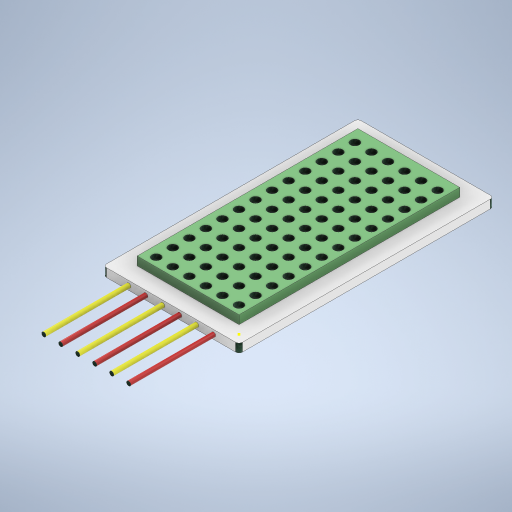
# Autodesk Inventor part: circuit
Saved by Autodesk Inventor 2024 (Build 280153000, 153)
## iProperties
Created: 2024-02-01
Part Number: circuit
Material: Generic
Document SubType Name: Modeling
Designer: RAHUL
Density: 1 g/cm^3
Appearance: Green Polished
Author: RAHUL
Autodesk Inventor part; units mm, degrees
ref_plane "YZ Plane" through (0, 0, 0) normal (1, 0, 0) x (0, 1, 0)
ref_plane "XZ Plane" through (0, 0, 0) normal (0, 1, 0) x (-1, 0, 0)
ref_plane "XY Plane" through (0, 0, 0) normal (0, 0, 1) x (1, 0, 0)
sketch "Sketch1" plane through (0, 0, 0) normal (0, 1, 0) x (-1, 0, 0)
  line L0 (0, 0) -> (80, 0)
  line L1 (80, 0) -> (80, -150)
  line L2 (80, -150) -> (0, -150)
  line L3 (0, -150) -> (0, 0)
  dimension "d0" = 80
  dimension "d1" = 150
  constraints: 8 end point, 2 parallel, 1 horizontal, 1 perpendicular
  measures "d0" distance of L1.end L2.end
  measures "d1" distance of L0.end L1.end
extrude "Extrusion1" add sketch "Sketch1" against normal blind 5
fillet "Fillet1" radius 2 4 edges at (0, -2.5, 0) (0, -2.5, -150) (-80, -2.5, 0) (-80, -2.5, -150)
sketch "Sketch2" plane through (0, 0, 0) normal (0, 1, 0) x (1, 0, 0)
  line L0 (-70, 140) -> (-10, 140)
  line L1 (-10, 140) -> (-10, 10)
  line L2 (-10, 10) -> (-70, 10)
  line L3 (-70, 10) -> (-70, 140)
  line L4 (-2, 150) -> (-78, 150) projected
  line L5 (0, 2) -> (0, 148) projected
  line L6 (-80, 148) -> (-80, 2) projected
  point P0 (0, 0)
  dimension "d5" = 10
  dimension "d6" = 10
  dimension "d7" = 10
  dimension "d8" = 10
  constraints: 8 end point, 2 parallel, 1 horizontal, 1 perpendicular
  measures "d5" distance between parallel lines of L4 L0
  measures "d6" distance from line of point (0, 0) L2
  measures "d7" distance between parallel lines of L5 L1
  measures "d8" distance between parallel lines of L6 L3
extrude "Extrusion2" add sketch "Sketch2" along normal blind 5
sketch "Sketch3" plane through (0, 5, 0) normal (0, 1, 0) x (1, 0, 0)
  point P0 (0, 0)
sketch "Sketch5" plane through (0, 5, 0) normal (0, 1, 0) x (1, 0, 0)
  circle A0 centre (-15, 15) radius 2.5
  line L0 (-70, 10) -> (-10, 10) projected
  line L1 (-10, 10) -> (-10, 140) projected
  point P0 (0, 0)
  dimension "d11" = 5
  dimension "d12" = 5
  dimension "d13" = 5
  constraints: 1 centre point
  measures "d11" diameter of A0
  measures "d12" distance from line of L0 A0.centre
  measures "d13" distance from line of L1 A0.centre
extrude "Extrusion3" cut sketch "Sketch5" against normal blind 3
pattern_linear "Rectangular Pattern1" count 6 spacing -9.75 along (1, 0, 0) count 13 spacing 9.75 along (0, 0, -1) of "Extrusion3"
sketch "Sketch6" plane through (-78, 0, 0) normal (0, 0, 1) x (1, 0, 0)
  circle A0 centre (63, -2.5) radius 1.25
  line L0 (0, 0) -> (76, 0) projected
  line L1 (78, -5) -> (78, 0) projected
  dimension "d22" = 2.5
  dimension "d23" = 2.5
  dimension "d24" = 15
  constraints: 1 centre point
  measures "d22" diameter of A0
  measures "d23" distance from line of L0 A0.centre
  measures "d24" distance from line of L1 A0.centre
extrude "Extrusion4" add sketch "Sketch6" along normal blind 50
pattern_linear "Rectangular Pattern2" count 6 spacing -10 along (1, 0, 0) of "Extrusion4"
body "Solid1"
